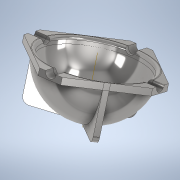
# Autodesk Inventor part: Stewart Boogert Ash Tray
Saved by Autodesk Inventor 2020.2 (Build 242310000, 310)
## iProperties
Created: 2019-12-18
Part Number: Stewart Boogert Ash Tray
Material: Generic
Document SubType Name: Modeling
Designer: uwap015
Density: 1 g/cm^3
Appearance: Steel - Polished
Author: uwap015
Autodesk Inventor part; units mm, degrees
sketch "Sketch1" plane through (0, 0, 0) normal (0, 1, 0) x (-1, 0, 0)
  arc A0 (40, 0) -> (0, 40) centre (0, 0) ccw
  line L0 (0, 40) -> (0, 0)
  line L1 (0, 0) -> (40, 0)
  line L2 (0, -9.6569) -> (0, 57.9411) projected
  constraints: 4 end point, 2 point on circle, 1 centre point, 1 coincident, 1 perpendicular, 1 vertical
revolve "Revolution1" add sketch "Sketch1" angle 360 about axis through (0, 0, -10) along (0, 0, 1)
ref_plane "Work Plane1" through (0, 40, 0) normal (0, 1, 0) x (-1, 0, 0)
ref_plane "Work Plane2" through (0, 0, 40) normal (0, 0, 1) x (1, 0, 0)
ref_plane "Work Plane3" through (0, 0, 40) normal (0, 0, 1) x (1, 0, 0)
sketch "Sketch9" plane through (0, 0, 40) normal (0, 0, 1) x (1, 0, 0)
  line L0 (0, 0) -> (46.188, 0) construction
  line L1 (0, 0) -> (46.188, 0) construction
  line L2 (-2, 1.1547) -> (-2, 40)
  line L3 (2, 1.1547) -> (2, 40)
  line L4 (2, 1.1547) -> (35.641, -18.2679)
  line L5 (0, -2.3094) -> (33.641, -21.7321)
  line L6 (-2, 1.1547) -> (-35.641, -18.2679)
  line L7 (0, -2.3094) -> (-33.641, -21.7321)
  line L8 (-2, 40) -> (2, 40)
  line L9 (35.641, -18.2679) -> (33.641, -21.7321)
  line L10 (-35.641, -18.2679) -> (-33.641, -21.7321)
  constraints: 22 end point, 2 horizontal, 2 perpendicular
extrude "Extrusion3" add sketch "Sketch9" against normal blind 40
sketch "Sketch10" plane through (0, 0, 0) normal (0, 0, -1) x (-1, 0, 0)
  line L0 (40, -40) -> (-40, -40)
  line L1 (-40, -40) -> (-40, 40)
  line L2 (-40, 40) -> (40, 40)
  line L3 (40, 40) -> (40, -40)
  line L4 (40, -40) -> (-40, 40) construction
  line L5 (-40, -40) -> (40, 40) construction
  point P0 (0, 0)
  constraints: 12 end point, 2 midpoint, 2 parallel, 1 horizontal, 1 perpendicular
extrude "Extrusion4" add sketch "Sketch10" against normal blind 5 separate body
sketch "Sketch12" plane through (0, 0, 0) normal (0, 1, 0) x (-1, 0, 0)
  arc A0 (37, 0) -> (0, 37) centre (0, 0) ccw
  line L0 (-40, 0) -> (40, 0) projected
  line L1 (37, 0) -> (0, 0)
  line L2 (0, 0) -> (0, 37)
  line L3 (0, -8.9326) -> (0, 53.5955) projected
  dimension "d42" = 37
  constraints: 4 end point, 2 point on circle, 1 centre point, 1 coincident, 1 collinear, 1 perpendicular, 1 point on line
  measures "d42" radius of A0
revolve "Revolution3" cut sketch "Sketch12" angle 360 about axis through (0, 0, -10) along (0, 0, 1) bodies 2 1
chamfer "Chamfer1" distance 12 angle 45 4 edges at (-40, 40, 2.5) (40, 40, 2.5) (40, -40, 2.5) (-40, -40, 2.5)
fillet "Fillet3" radius 2.5 1 edges at (37, 0, 0)
fillet "Fillet4" radius 5 3 edges at (34.641, -20, 40) (0, 40, 40) (-34.641, -20, 40)
sketch "Sketch13" plane through (-28, 40, 0) normal (-0.7071, 0.7071, 0) x (-0.7071, -0.7071, 0)
  arc A0 (12.4853, 0) -> (4.4853, 0) centre (8.4853, 0) ccw
  line L0 (-18.3494, 0) -> (46.5563, 0) projected
  line L1 (12.4853, 0) -> (4.4853, 0)
  dimension "d51" = 8
  constraints: 2 end point, 2 point on circle, 2 point on line, 1 centre point, 1 coincident
  measures "d51" diameter of A0
extrude "Extrusion6" cut sketch "Sketch13" against normal through all bodies 2 1
sketch "Sketch14" plane through (40, 28, 0) normal (0.7071, 0.7071, 0) x (-0.7071, 0.7071, 0)
  arc A0 (12.4853, 0) -> (4.4853, 0) centre (8.4853, 0) ccw
  line L0 (-29.5858, 0) -> (35.32, 0) projected
  line L1 (4.4853, 0) -> (12.4853, 0)
  dimension "d56" = 8
  constraints: 2 end point, 2 point on circle, 2 point on line, 1 centre point, 1 coincident
  measures "d56" diameter of A0
extrude "Extrusion7" cut sketch "Sketch14" against normal through all bodies 2 1
body "Solid1"
body "Solid2"
